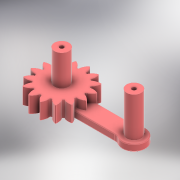
# Autodesk Inventor part: BRAÇO ROBÓTICO - Garra A2a
Saved by Autodesk Inventor 2021 (Build 250183000, 183)
## iProperties
Created: 2020-08-23
Part Number: BRAÇO ROBÓTICO - Garra A2a
Material: Plástico PC/ABS
Document SubType Name: Modeling
Designer: Araújo, I.
Density: 0.357273 g/cm^3
Appearance: Liso - Branco
Mass: 0.693061 g
Surface Area: 18.6744 cm^2
Volume: 1.93987 cm^3
Author: Araújo, I.
## iProperties of the stored document _3DPrint.ipt
Created: 2020-11-23
Part Number: _3DPrint
Material: Genérico
Document SubType Name: Modeling
Designer: Araújo, I.
Mass: 1.93987 g
Surface Area: 18.6744 cm^2
Volume: 1.93987 cm^3
Density: 1 g/cm^3
Appearance: Padrão
Author: Araújo, I.
Autodesk Inventor part; units mm, degrees
ref_plane "YZ Plane" through (0, 0, 0) normal (1, 0, 0) x (0, 1, 0)
ref_plane "XZ Plane" through (0, 0, 0) normal (0, 1, 0) x (-1, 0, 0)
ref_plane "XY Plane" through (0, 0, 0) normal (0, 0, 1) x (1, 0, 0)
sketch "Esboço2" plane through (0, 0, 0) normal (0, 1, 0) x (-1, 0, 0)
  arc A0 (-2.0603, -3.4286) -> (-2.0603, 3.4286) centre (0, 0) ccw
  arc A1 (-22.9397, 3.4286) -> (-22.9397, -3.4286) centre (-25, 0) ccw
  line L0 (-3.6056, -3) -> (-21.3944, -3)
  line L1 (-3.6056, 3) -> (-21.3944, 3)
  arc A2 (-2.0603, -3.4286) -> (-3.6056, -3) centre (-3.6056, -6) ccw
  arc A3 (-3.6056, 3) -> (-2.0603, 3.4286) centre (-3.6056, 6) ccw
  arc A4 (-21.3944, -3) -> (-22.9397, -3.4286) centre (-21.3944, -6) ccw
  arc A5 (-22.9397, 3.4286) -> (-21.3944, 3) centre (-21.3944, 6) ccw
  dimension "d64" = 6
  dimension "d65" = 3
  dimension "d94" = 25
  dimension "d95" = 4
  constraints: 12 point on circle, 8 tangent, 6 centre point, 4 end point, 4 equal radius, 2 parallel, 1 coincident, 1 horizontal, 1 horizontal alignment
  measures "d64" distance between parallel lines of L1 L0
  measures "d65" radius of A2
  measures "d94" distance of A1.centre A0.centre
  measures "d95" radius of A0
extrude "Extrusão2" add sketch "Esboço2" along normal blind 2.5
fillet "Arredondamento2" radius 0.3 16 edges at (22.1962, 2.5, 3.1091) (29, 2.5, 0) (22.1962, 2.5, -3.1091) (12.5, 2.5, -3) (2.8038, 2.5, -3.1091) (-4, 2.5, 0) (2.8038, 2.5, 3.1091) (12.5, 2.5, 3) (22.1962, 0, 3.1091) (29, 0, 0) (22.1962, 0, -3.1091) (12.5, 0, -3) (2.8038, 0, -3.1091) (-4, 0, 0) (2.8038, 0, 3.1091) (12.5, 0, 3)
sketch "Esboço1" plane through (0, 0, 0) normal (0, 1, 0) x (-1, 0, 0)
  circle A0 centre (0, 0) radius 8.5 construction
  line L0 (-16.1333, -15) -> (-23.1333, -15) construction
  line L1 (-23.1333, -15) -> (-23.1333, -7) construction
  line L2 (-23.1333, -7) -> (-16.1333, -7) construction
  line L3 (-16.1333, -7) -> (-16.1333, -15) construction
  circle A1 centre (0, 0) radius 9.6333
  circle A2 centre (0, 0) radius 7.3667 construction
  circle A3 centre (0, 0) radius 7.1778 construction
  line L4 (0, -15) -> (-1.1333, -15) construction
  line L5 (0, 0) -> (0, -9.6333)
  arc A4 (1.1679, -7.3143) -> (1.1647, -7.274) centre (0.3979, -7.3559) ccw construction
  line L6 (1.1647, -7.274) -> (0, 0) construction
  line L7 (0, 0) -> (0.3979, -7.3559) construction
  line L8 (0, 0) -> (-0.3731, -7.3572) construction
  line L9 (0, 0) -> (-1.1401, -7.2779) construction
  line L10 (0, 0) -> (-1.8946, -7.1189) construction
  line L11 (0, 0) -> (-2.6284, -6.8818) construction
  line L12 (1.1679, -7.3143) -> (0.3979, -7.3559) construction
  arc A5 (1.1665, -7.4353) -> (1.1679, -7.3143) centre (-0.3731, -7.3572) ccw construction
  line L13 (1.1665, -7.4353) -> (-0.3731, -7.3572) construction
  arc A6 (1.144, -7.6357) -> (1.1665, -7.4353) centre (-1.1401, -7.2779) ccw construction
  line L14 (1.144, -7.6357) -> (-1.1401, -7.2779) construction
  line L15 (-1.8946, -7.1189) -> (1.084, -7.9116) construction
  line L16 (-2.6284, -6.8818) -> (0.9706, -8.2564) construction
  arc A7 (1.084, -7.9116) -> (1.144, -7.6357) centre (-1.8946, -7.1189) ccw construction
  arc A8 (0.9706, -8.2564) -> (1.084, -7.9116) centre (-2.6284, -6.8818) ccw construction
  line L17 (0, 0) -> (-3.3333, -6.5694) construction
  line L18 (0, 0) -> (-4.0018, -6.185) construction
  line L19 (0, 0) -> (-4.6263, -5.7328) construction
  line L20 (-3.3333, -6.5694) -> (0.7891, -8.6611) construction
  line L21 (-4.0018, -6.185) -> (0.5261, -9.1145) construction
  line L22 (-4.6263, -5.7328) -> (0.1698, -9.6033) construction
  arc A9 (0.7891, -8.6611) -> (0.9706, -8.2564) centre (-3.3333, -6.5694) ccw construction
  arc A10 (0.5261, -9.1145) -> (0.7891, -8.6611) centre (-4.0018, -6.185) ccw construction
  arc A11 (0.1698, -9.6033) -> (0.5261, -9.1145) centre (-4.6263, -5.7328) ccw construction
  line L23 (0, 0) -> (-5.2002, -5.2178) construction
  line L24 (-5.2002, -5.2178) -> (-0.2895, -10.1121) construction
  arc A12 (-0.2895, -10.1121) -> (0.1698, -9.6033) centre (-5.2002, -5.2178) ccw construction
  line L25 (0, 0) -> (-5.7172, -4.6456) construction
  line L26 (-5.7172, -4.6456) -> (-0.8592, -10.6241) construction
  arc A13 (-0.8592, -10.6241) -> (-0.2895, -10.1121) centre (-5.7172, -4.6456) ccw construction
  spline S0 degree 4 poles (1.1647, -7.274) (1.1686, -7.2985) (1.1736, -7.4195) (1.154, -7.6223) (1.0788, -7.957) (0.9627, -8.2995) (0.7787, -8.7043) (0.3958, -9.356) (-0.0581, -9.9105) (-0.4987, -10.3319) (-0.8592, -10.6241) knots 0 0 0 0 0 0.136483 0.216899 0.310564 0.415677 0.531051 0.655814 1 1 1 1 1
  line L27 (0, 0) -> (0.8885, -8.4534) construction
  line L28 (0, -19.8966) -> (0, 14.3795) projected
  line L29 (-1.1333, -15) -> (-16.1333, -15) construction
  spline S1 degree 4 poles (-1.1647, -7.274) (-1.1686, -7.2985) (-1.1736, -7.4195) (-1.154, -7.6223) (-1.0788, -7.957) (-0.9627, -8.2995) (-0.7787, -8.7043) (-0.3958, -9.356) (0.0581, -9.9105) (0.4987, -10.3319) (0.8592, -10.6241) knots 0 0 0 0 0 0.136483 0.216899 0.310564 0.415677 0.531051 0.655814 1 1 1 1 1
  arc A14 (-1.6676, -6.9814) -> (-1.3161, -7.0561) centre (0, 0) ccw
  arc A15 (-1.1647, -7.274) -> (-1.3161, -7.0561) centre (-1.3508, -7.2418) ccw
  arc A16 (-1.6676, -6.9814) -> (-1.8946, -7.1189) centre (-1.7115, -7.1651) ccw
  spline S2 degree 4 poles (4.0226, -6.1714) (4.0362, -6.1922) (4.0899, -6.3007) (4.1545, -6.4939) (4.2219, -6.8302) (4.2552, -7.1904) (4.2517, -7.6351) (4.1671, -8.3862) (3.9779, -9.0773) (3.7468, -9.6415) (3.5363, -10.0551) knots 0 0 0 0 0 0.136483 0.216899 0.310564 0.415677 0.531051 0.655814 1 1 1 1 1
  spline S3 degree 4 poles (1.8946, -7.1189) (1.9009, -7.1428) (1.9457, -7.2554) (2.046, -7.4327) (2.2508, -7.7078) (2.4962, -7.9736) (2.829, -8.2685) (3.4438, -8.7082) (4.084, -9.03) (4.6579, -9.2358) (5.1061, -9.3561) knots 0 0 0 0 0 0.136483 0.216899 0.310564 0.415677 0.531051 0.655814 1 1 1 1 1
  spline S4 degree 4 poles (6.185, -4.0018) (6.2058, -4.0152) (6.2991, -4.0925) (6.4366, -4.2427) (6.635, -4.5225) (6.8119, -4.838) (6.9896, -5.2457) (7.2178, -5.9663) (7.326, -6.6746) (7.3444, -7.284) (7.3203, -7.7474) knots 0 0 0 0 0 0.136483 0.216899 0.310564 0.415677 0.531051 0.655814 1 1 1 1 1
  spline S5 degree 4 poles (4.6263, -5.7328) (4.6418, -5.7521) (4.7285, -5.8368) (4.8923, -5.9579) (5.1913, -6.126) (5.5236, -6.2689) (5.9475, -6.403) (6.688, -6.5546) (7.4038, -6.5882) (8.0118, -6.5428) (8.4702, -6.4704) knots 0 0 0 0 0 0.136483 0.216899 0.310564 0.415677 0.531051 0.655814 1 1 1 1 1
  spline S6 degree 4 poles (7.2779, -1.1401) (7.3024, -1.1439) (7.419, -1.1766) (7.6058, -1.2579) (7.9009, -1.4328) (8.1908, -1.6491) (8.5189, -1.9492) (9.0204, -2.5147) (9.4075, -3.1177) (9.6721, -3.667) (9.8386, -4.1002) knots 0 0 0 0 0 0.136483 0.216899 0.310564 0.415677 0.531051 0.655814 1 1 1 1 1
  spline S7 degree 4 poles (6.5581, -3.3554) (6.5801, -3.3668) (6.6937, -3.4089) (6.8926, -3.4529) (7.2341, -3.4849) (7.5958, -3.4803) (8.0377, -3.4303) (8.7758, -3.2676) (9.4434, -3.0073) (9.9803, -2.7184) (10.3696, -2.4659) knots 0 0 0 0 0 0.136483 0.216899 0.310564 0.415677 0.531051 0.655814 1 1 1 1 1
  spline S8 degree 4 poles (7.1124, 1.9186) (7.1363, 1.9251) (7.2562, 1.9427) (7.4599, 1.9444) (7.8006, 1.9046) (8.1534, 1.825) (8.5752, 1.6842) (9.2634, 1.3716) (9.8622, 0.9782) (10.3274, 0.584) (10.6557, 0.256) knots 0 0 0 0 0 0.136483 0.216899 0.310564 0.415677 0.531051 0.655814 1 1 1 1 1
  spline S9 degree 4 poles (7.3559, -0.3979) (7.3806, -0.3993) (7.5015, -0.3916) (7.7011, -0.3509) (8.0261, -0.2412) (8.3547, -0.0899) (8.738, 0.1355) (9.3462, 0.5843) (9.8501, 1.0937) (10.2232, 1.5759) (10.4761, 1.965) knots 0 0 0 0 0 0.136483 0.216899 0.310564 0.415677 0.531051 0.655814 1 1 1 1 1
  spline S10 degree 4 poles (5.7172, 4.6456) (5.7363, 4.6613) (5.8387, 4.7261) (6.0241, 4.8105) (6.3515, 4.9128) (6.7062, 4.9835) (7.1488, 5.0265) (7.9047, 5.0208) (8.6118, 4.9049) (9.197, 4.7341) (9.6303, 4.568) knots 0 0 0 0 0 0.136483 0.216899 0.310564 0.415677 0.531051 0.655814 1 1 1 1 1
  spline S11 degree 4 poles (6.8818, 2.6284) (6.905, 2.6372) (7.0123, 2.6934) (7.1781, 2.8117) (7.4303, 3.0442) (7.669, 3.316) (7.9275, 3.6778) (8.3005, 4.3352) (8.5537, 5.0055) (8.6983, 5.5978) (8.7711, 6.0561) knots 0 0 0 0 0 0.136483 0.216899 0.310564 0.415677 0.531051 0.655814 1 1 1 1 1
  spline S12 degree 4 poles (3.3333, 6.5694) (3.3445, 6.5915) (3.4116, 6.6923) (3.5467, 6.8448) (3.8042, 7.0714) (4.0995, 7.2803) (4.4863, 7.4996) (5.1791, 7.8019) (5.8722, 7.9836) (6.4764, 8.0656) (6.9398, 8.09) knots 0 0 0 0 0 0.136483 0.216899 0.310564 0.415677 0.531051 0.655814 1 1 1 1 1
  spline S13 degree 4 poles (5.2178, 5.2002) (5.2354, 5.2177) (5.3105, 5.3127) (5.4139, 5.4882) (5.5498, 5.8032) (5.6572, 6.1486) (5.7462, 6.5842) (5.8196, 7.3365) (5.7782, 8.0519) (5.6695, 8.6518) (5.5496, 9.1001) knots 0 0 0 0 0 0.136483 0.216899 0.310564 0.415677 0.531051 0.655814 1 1 1 1 1
  spline S14 degree 4 poles (0.3731, 7.3572) (0.3743, 7.382) (0.3947, 7.5014) (0.456, 7.6956) (0.5991, 8.0074) (0.7839, 8.3183) (1.0481, 8.676) (1.5581, 9.2339) (2.1173, 9.6818) (2.6359, 10.0024) (3.0493, 10.2133) knots 0 0 0 0 0 0.136483 0.216899 0.310564 0.415677 0.531051 0.655814 1 1 1 1 1
  spline S15 degree 4 poles (2.6516, 6.8729) (2.6605, 6.896) (2.6905, 7.0134) (2.7135, 7.2158) (2.7096, 7.5588) (2.6672, 7.918) (2.5714, 8.3522) (2.3324, 9.0693) (2.0037, 9.706) (1.6603, 10.2098) (1.3684, 10.5706) knots 0 0 0 0 0 0.136483 0.216899 0.310564 0.415677 0.531051 0.655814 1 1 1 1 1
  spline S16 degree 4 poles (-2.6516, 6.8729) (-2.6605, 6.896) (-2.6905, 7.0134) (-2.7135, 7.2158) (-2.7096, 7.5588) (-2.6672, 7.918) (-2.5714, 8.3522) (-2.3324, 9.0693) (-2.0037, 9.706) (-1.6603, 10.2098) (-1.3684, 10.5706) knots 0 0 0 0 0 0.136483 0.216899 0.310564 0.415677 0.531051 0.655814 1 1 1 1 1
  spline S17 degree 4 poles (-0.3731, 7.3572) (-0.3743, 7.382) (-0.3947, 7.5014) (-0.456, 7.6956) (-0.5991, 8.0074) (-0.7839, 8.3183) (-1.0481, 8.676) (-1.5581, 9.2339) (-2.1173, 9.6818) (-2.6359, 10.0024) (-3.0493, 10.2133) knots 0 0 0 0 0 0.136483 0.216899 0.310564 0.415677 0.531051 0.655814 1 1 1 1 1
  spline S18 degree 4 poles (-5.2178, 5.2002) (-5.2354, 5.2177) (-5.3105, 5.3127) (-5.4139, 5.4882) (-5.5498, 5.8032) (-5.6572, 6.1486) (-5.7462, 6.5842) (-5.8196, 7.3365) (-5.7782, 8.0519) (-5.6695, 8.6518) (-5.5496, 9.1001) knots 0 0 0 0 0 0.136483 0.216899 0.310564 0.415677 0.531051 0.655814 1 1 1 1 1
  spline S19 degree 4 poles (-3.3333, 6.5694) (-3.3445, 6.5915) (-3.4116, 6.6923) (-3.5467, 6.8448) (-3.8042, 7.0714) (-4.0995, 7.2803) (-4.4863, 7.4996) (-5.1791, 7.8019) (-5.8722, 7.9836) (-6.4764, 8.0656) (-6.9398, 8.09) knots 0 0 0 0 0 0.136483 0.216899 0.310564 0.415677 0.531051 0.655814 1 1 1 1 1
  spline S20 degree 4 poles (-6.8818, 2.6284) (-6.905, 2.6372) (-7.0123, 2.6934) (-7.1781, 2.8117) (-7.4303, 3.0442) (-7.669, 3.316) (-7.9275, 3.6778) (-8.3005, 4.3352) (-8.5537, 5.0055) (-8.6983, 5.5978) (-8.7711, 6.0561) knots 0 0 0 0 0 0.136483 0.216899 0.310564 0.415677 0.531051 0.655814 1 1 1 1 1
  spline S21 degree 4 poles (-5.7172, 4.6456) (-5.7363, 4.6613) (-5.8387, 4.7261) (-6.0241, 4.8105) (-6.3515, 4.9128) (-6.7062, 4.9835) (-7.1488, 5.0265) (-7.9047, 5.0208) (-8.6118, 4.9049) (-9.197, 4.7341) (-9.6303, 4.568) knots 0 0 0 0 0 0.136483 0.216899 0.310564 0.415677 0.531051 0.655814 1 1 1 1 1
  spline S22 degree 4 poles (-7.3559, -0.3979) (-7.3806, -0.3993) (-7.5015, -0.3916) (-7.7011, -0.3509) (-8.0261, -0.2412) (-8.3547, -0.0899) (-8.738, 0.1355) (-9.3462, 0.5843) (-9.8501, 1.0937) (-10.2232, 1.5759) (-10.4761, 1.965) knots 0 0 0 0 0 0.136483 0.216899 0.310564 0.415677 0.531051 0.655814 1 1 1 1 1
  spline S23 degree 4 poles (-7.1124, 1.9186) (-7.1363, 1.9251) (-7.2562, 1.9427) (-7.4599, 1.9444) (-7.8006, 1.9046) (-8.1534, 1.825) (-8.5752, 1.6842) (-9.2634, 1.3716) (-9.8622, 0.9782) (-10.3274, 0.584) (-10.6557, 0.256) knots 0 0 0 0 0 0.136483 0.216899 0.310564 0.415677 0.531051 0.655814 1 1 1 1 1
  spline S24 degree 4 poles (-6.5581, -3.3554) (-6.5801, -3.3668) (-6.6937, -3.4089) (-6.8926, -3.4529) (-7.2341, -3.4849) (-7.5958, -3.4803) (-8.0377, -3.4303) (-8.7758, -3.2676) (-9.4434, -3.0073) (-9.9803, -2.7184) (-10.3696, -2.4659) knots 0 0 0 0 0 0.136483 0.216899 0.310564 0.415677 0.531051 0.655814 1 1 1 1 1
  spline S25 degree 4 poles (-7.2779, -1.1401) (-7.3024, -1.1439) (-7.419, -1.1766) (-7.6058, -1.2579) (-7.9009, -1.4328) (-8.1908, -1.6491) (-8.5189, -1.9492) (-9.0204, -2.5147) (-9.4075, -3.1177) (-9.6721, -3.667) (-9.8386, -4.1002) knots 0 0 0 0 0 0.136483 0.216899 0.310564 0.415677 0.531051 0.655814 1 1 1 1 1
  spline S26 degree 4 poles (-4.6263, -5.7328) (-4.6418, -5.7521) (-4.7285, -5.8368) (-4.8923, -5.9579) (-5.1913, -6.126) (-5.5236, -6.2689) (-5.9475, -6.403) (-6.688, -6.5546) (-7.4038, -6.5882) (-8.0118, -6.5428) (-8.4702, -6.4704) knots 0 0 0 0 0 0.136483 0.216899 0.310564 0.415677 0.531051 0.655814 1 1 1 1 1
  spline S27 degree 4 poles (-6.185, -4.0018) (-6.2058, -4.0152) (-6.2991, -4.0925) (-6.4366, -4.2427) (-6.635, -4.5225) (-6.8119, -4.838) (-6.9896, -5.2457) (-7.2178, -5.9663) (-7.326, -6.6746) (-7.3444, -7.284) (-7.3203, -7.7474) knots 0 0 0 0 0 0.136483 0.216899 0.310564 0.415677 0.531051 0.655814 1 1 1 1 1
  spline S28 degree 4 poles (-1.8946, -7.1189) (-1.9009, -7.1428) (-1.9457, -7.2554) (-2.046, -7.4327) (-2.2508, -7.7078) (-2.4962, -7.9736) (-2.829, -8.2685) (-3.4438, -8.7082) (-4.084, -9.03) (-4.6579, -9.2358) (-5.1061, -9.3561) knots 0 0 0 0 0 0.136483 0.216899 0.310564 0.415677 0.531051 0.655814 1 1 1 1 1
  spline S29 degree 4 poles (-4.0226, -6.1714) (-4.0362, -6.1922) (-4.0899, -6.3007) (-4.1545, -6.4939) (-4.2219, -6.8302) (-4.2552, -7.1904) (-4.2517, -7.6351) (-4.1671, -8.3862) (-3.9779, -9.0773) (-3.7468, -9.6415) (-3.5363, -10.0551) knots 0 0 0 0 0 0.136483 0.216899 0.310564 0.415677 0.531051 0.655814 1 1 1 1 1
  arc A17 (1.8946, -7.1189) -> (1.6676, -6.9814) centre (1.7115, -7.1651) ccw
  arc A18 (1.3161, -7.0561) -> (1.6676, -6.9814) centre (0, 0) ccw
  arc A19 (1.3161, -7.0561) -> (1.1647, -7.274) centre (1.3508, -7.2418) ccw
  arc A20 (4.6263, -5.7328) -> (4.363, -5.6995) centre (4.4778, -5.8495) ccw
  arc A21 (4.0723, -5.9107) -> (4.363, -5.6995) centre (0, 0) ccw
  arc A22 (4.0723, -5.9107) -> (4.0226, -6.1714) centre (4.1795, -6.0663) ccw
  arc A23 (6.5581, -3.3554) -> (6.304, -3.4322) centre (6.4699, -3.5225) ccw
  arc A24 (6.1244, -3.7434) -> (6.304, -3.4322) centre (0, 0) ccw
  arc A25 (6.1244, -3.7434) -> (6.185, -4.0018) centre (6.2855, -3.8419) ccw
  arc A26 (7.3559, -0.3979) -> (7.155, -0.5714) centre (7.3433, -0.5864) ccw
  arc A27 (7.1174, -0.9287) -> (7.155, -0.5714) centre (0, 0) ccw
  arc A28 (7.1174, -0.9287) -> (7.2779, -1.1401) centre (7.3047, -0.9532) ccw
  arc A29 (6.8818, 2.6284) -> (6.7688, 2.3882) centre (6.9469, 2.4511) ccw
  arc A30 (6.8799, 2.0465) -> (6.7688, 2.3882) centre (0, 0) ccw
  arc A31 (6.8799, 2.0465) -> (7.1124, 1.9186) centre (7.0609, 2.1003) ccw
  arc A32 (5.2178, 5.2002) -> (5.2122, 4.9349) centre (5.3494, 5.0648) ccw
  arc A33 (5.4527, 4.6678) -> (5.2122, 4.9349) centre (0, 0) ccw
  arc A34 (5.4527, 4.6678) -> (5.7172, 4.6456) centre (5.5962, 4.7907) ccw
  arc A35 (2.6516, 6.8729) -> (2.7544, 6.6282) centre (2.8269, 6.8027) ccw
  arc A36 (3.0827, 6.4821) -> (2.7544, 6.6282) centre (0, 0) ccw
  arc A37 (3.0827, 6.4821) -> (3.3333, 6.5694) centre (3.1638, 6.6527) ccw
  arc A38 (-0.3731, 7.3572) -> (-0.1797, 7.1755) centre (-0.1844, 7.3644) ccw
  arc A39 (0.1797, 7.1755) -> (-0.1797, 7.1755) centre (0, 0) ccw
  arc A40 (0.1797, 7.1755) -> (0.3731, 7.3572) centre (0.1844, 7.3644) ccw
  arc A41 (-3.3333, 6.5694) -> (-3.0827, 6.4821) centre (-3.1638, 6.6527) ccw
  arc A42 (-2.7544, 6.6282) -> (-3.0827, 6.4821) centre (0, 0) ccw
  arc A43 (-2.7544, 6.6282) -> (-2.6516, 6.8729) centre (-2.8269, 6.8027) ccw
  arc A44 (-5.7172, 4.6456) -> (-5.4527, 4.6678) centre (-5.5962, 4.7907) ccw
  arc A45 (-5.2122, 4.9349) -> (-5.4527, 4.6678) centre (0, 0) ccw
  arc A46 (-5.2122, 4.9349) -> (-5.2178, 5.2002) centre (-5.3494, 5.0648) ccw
  arc A47 (-7.1124, 1.9186) -> (-6.8799, 2.0465) centre (-7.0609, 2.1003) ccw
  arc A48 (-6.7688, 2.3882) -> (-6.8799, 2.0465) centre (0, 0) ccw
  arc A49 (-6.7688, 2.3882) -> (-6.8818, 2.6284) centre (-6.9469, 2.4511) ccw
  arc A50 (-7.2779, -1.1401) -> (-7.1174, -0.9287) centre (-7.3047, -0.9532) ccw
  arc A51 (-7.155, -0.5714) -> (-7.1174, -0.9287) centre (0, 0) ccw
  arc A52 (-7.155, -0.5714) -> (-7.3559, -0.3979) centre (-7.3433, -0.5864) ccw
  arc A53 (-6.185, -4.0018) -> (-6.1244, -3.7434) centre (-6.2855, -3.8419) ccw
  arc A54 (-6.304, -3.4322) -> (-6.1244, -3.7434) centre (0, 0) ccw
  arc A55 (-6.304, -3.4322) -> (-6.5581, -3.3554) centre (-6.4699, -3.5225) ccw
  arc A56 (-4.0226, -6.1714) -> (-4.0723, -5.9107) centre (-4.1795, -6.0663) ccw
  arc A57 (-4.363, -5.6995) -> (-4.0723, -5.9107) centre (0, 0) ccw
  arc A58 (-4.363, -5.6995) -> (-4.6263, -5.7328) centre (-4.4778, -5.8495) ccw
  point P0 (-1.1679, -7.3143)
  point P1 (-1.1665, -7.4353)
  point P2 (-1.144, -7.6357)
  point P3 (-1.084, -7.9116)
  point P4 (-0.9706, -8.2564)
  point P5 (-0.7891, -8.6611)
  point P6 (-0.5261, -9.1145)
  point P7 (-0.1698, -9.6033)
  point P8 (0.2895, -10.1121)
  point P9 (-0.1462, -9.6322)
  point P10 (0.1462, -9.6322)
  point P11 (4.0419, -6.2069)
  point P12 (4.0899, -6.318)
  point P13 (4.1508, -6.5103)
  point P14 (4.2082, -6.7867)
  point P15 (4.2449, -7.1478)
  point P16 (4.2437, -7.5914)
  point P17 (4.1878, -8.1126)
  point P18 (4.0611, -8.7039)
  point P19 (3.8485, -9.3556)
  point P20 (4.25, -7.3612)
  point P21 (1.9081, -7.1569)
  point P22 (1.9585, -7.2669)
  point P23 (2.0606, -7.4409)
  point P24 (2.2277, -7.6685)
  point P25 (2.4715, -7.9374)
  point P26 (2.8019, -8.2333)
  point P27 (3.2266, -8.5405)
  point P28 (3.7509, -8.8421)
  point P29 (4.3774, -9.1201)
  point P30 (6.217, -4.0263)
  point P31 (6.3061, -4.1083)
  point P32 (6.44, -4.2591)
  point P33 (6.6048, -4.4883)
  point P34 (6.7851, -4.8033)
  point P35 (6.9645, -5.209)
  point P36 (7.1254, -5.7079)
  point P37 (7.2502, -6.2996)
  point P38 (7.321, -6.9814)
  point P39 (6.8766, -4.9962)
  point P40 (4.6541, -5.7621)
  point P41 (4.745, -5.8421)
  point P42 (4.909, -5.9595)
  point P43 (5.1541, -6.0994)
  point P44 (5.4862, -6.2459)
  point P45 (5.9085, -6.3818)
  point P46 (6.4214, -6.4898)
  point P47 (7.023, -6.552)
  point P48 (7.7084, -6.5512)
  point P49 (7.3172, -1.1495)
  point P50 (7.4319, -1.1882)
  point P51 (7.6155, -1.2715)
  point P52 (7.8593, -1.4139)
  point P53 (8.1522, -1.6283)
  point P54 (8.4811, -1.926)
  point P55 (8.831, -2.3162)
  point P56 (9.1857, -2.8061)
  point P57 (9.5277, -3.4001)
  point P58 (8.3143, -1.7672)
  point P59 (6.5954, -3.371)
  point P60 (6.7109, -3.4071)
  point P61 (6.9085, -3.4476)
  point P62 (7.1894, -3.4757)
  point P63 (7.5524, -3.4744)
  point P64 (7.9934, -3.4269)
  point P65 (8.5059, -3.3169)
  point P66 (9.0808, -3.1291)
  point P67 (9.7066, -2.8495)
  point P68 (7.1521, 1.926)
  point P69 (7.2726, 1.9373)
  point P70 (7.4743, 1.9359)
  point P71 (7.755, 1.905)
  point P72 (8.1097, 1.8283)
  point P73 (8.5312, 1.6901)
  point P74 (9.0096, 1.4759)
  point P75 (9.5329, 1.1727)
  point P76 (10.0869, 0.7691)
  point P77 (8.3143, 1.7672)
  point P78 (7.3963, -0.3969)
  point P79 (7.5165, -0.3829)
  point P80 (7.7135, -0.3396)
  point P81 (7.9816, -0.251)
  point P82 (8.3126, -0.1022)
  point P83 (8.6962, 0.1206)
  point P84 (9.1196, 0.4295)
  point P85 (9.5684, 0.8349)
  point P86 (10.0264, 1.3449)
  point P87 (5.7504, 4.6686)
  point P88 (5.8559, 4.7279)
  point P89 (6.0407, 4.8086)
  point P90 (6.3097, 4.8945)
  point P91 (6.6649, 4.9687)
  point P92 (7.1062, 5.0139)
  point P93 (7.6304, 5.0129)
  point P94 (8.2318, 4.9487)
  point P95 (8.902, 4.8054)
  point P96 (6.8766, 4.9962)
  point P97 (6.9183, 2.6457)
  point P98 (7.0224, 2.7074)
  point P99 (7.1847, 2.8271)
  point P100 (7.3936, 3.017)
  point P101 (7.6355, 3.2876)
  point P102 (7.8953, 3.6472)
  point P103 (8.1564, 4.1017)
  point P104 (8.4016, 4.6546)
  point P105 (8.6126, 5.3067)
  point P106 (3.3544, 6.6038)
  point P107 (3.4266, 6.7009)
  point P108 (3.5626, 6.8499)
  point P109 (3.7734, 7.0378)
  point P110 (4.0678, 7.2501)
  point P111 (4.4525, 7.4708)
  point P112 (4.9318, 7.683)
  point P113 (5.5073, 7.869)
  point P114 (6.1779, 8.0107)
  point P115 (4.25, 7.3612)
  point P116 (5.2441, 5.2309)
  point P117 (5.3141, 5.3296)
  point P118 (5.4137, 5.505)
  point P119 (5.5273, 5.7635)
  point P120 (5.6382, 6.1091)
  point P121 (5.7293, 6.5432)
  point P122 (5.783, 7.0646)
  point P123 (5.782, 7.6694)
  point P124 (5.7095, 8.351)
  point P125 (0.3784, 7.3972)
  point P126 (0.4049, 7.5154)
  point P127 (0.4685, 7.7067)
  point P128 (0.5846, 7.9641)
  point P129 (0.7672, 8.2778)
  point P130 (1.0289, 8.6359)
  point P131 (1.3804, 9.0247)
  point P132 (1.8305, 9.4287)
  point P133 (2.3855, 9.8309)
  point P134 (0.8885, 8.4534)
  point P135 (2.6631, 6.9116)
  point P136 (2.6869, 7.0303)
  point P137 (2.7066, 7.231)
  point P138 (2.7052, 7.5133)
  point P139 (2.666, 7.8742)
  point P140 (2.5726, 8.3078)
  point P141 (2.4096, 8.806)
  point P142 (2.1627, 9.3581)
  point P143 (1.8193, 9.9513)
  point P144 (-2.6631, 6.9116)
  point P145 (-2.6869, 7.0303)
  point P146 (-2.7066, 7.231)
  point P147 (-2.7052, 7.5133)
  point P148 (-2.666, 7.8742)
  point P149 (-2.5726, 8.3078)
  point P150 (-2.4096, 8.806)
  point P151 (-2.1627, 9.3581)
  point P152 (-1.8193, 9.9513)
  point P153 (-2.6266, 8.084)
  point P154 (-0.3784, 7.3972)
  point P155 (-0.4049, 7.5154)
  point P156 (-0.4685, 7.7067)
  point P157 (-0.5846, 7.9641)
  point P158 (-0.7672, 8.2778)
  point P159 (-1.0289, 8.6359)
  point P160 (-1.3804, 9.0247)
  point P161 (-1.8305, 9.4287)
  point P162 (-2.3855, 9.8309)
  point P163 (-5.2441, 5.2309)
  point P164 (-5.3141, 5.3296)
  point P165 (-5.4137, 5.505)
  point P166 (-5.5273, 5.7635)
  point P167 (-5.6382, 6.1091)
  point P168 (-5.7293, 6.5432)
  point P169 (-5.783, 7.0646)
  point P170 (-5.782, 7.6694)
  point P171 (-5.7095, 8.351)
  point P172 (-5.6876, 6.3167)
  point P173 (-3.3544, 6.6038)
  point P174 (-3.4266, 6.7009)
  point P175 (-3.5626, 6.8499)
  point P176 (-3.7734, 7.0378)
  point P177 (-4.0678, 7.2501)
  point P178 (-4.4525, 7.4708)
  point P179 (-4.9318, 7.683)
  point P180 (-5.5073, 7.869)
  point P181 (-6.1779, 8.0107)
  point P182 (-6.9183, 2.6457)
  point P183 (-7.0224, 2.7074)
  point P184 (-7.1847, 2.8271)
  point P185 (-7.3936, 3.017)
  point P186 (-7.6355, 3.2876)
  point P187 (-7.8953, 3.6472)
  point P188 (-8.1564, 4.1017)
  point P189 (-8.4016, 4.6546)
  point P190 (-8.6126, 5.3067)
  point P191 (-7.7651, 3.4573)
  point P192 (-5.7504, 4.6686)
  point P193 (-5.8559, 4.7279)
  point P194 (-6.0407, 4.8086)
  point P195 (-6.3097, 4.8945)
  point P196 (-6.6649, 4.9687)
  point P197 (-7.1062, 5.0139)
  point P198 (-7.6304, 5.0129)
  point P199 (-8.2318, 4.9487)
  dimension "d13" = 17
  dimension "d23" = 19.2667
  dimension "d25" = 14.7333
  dimension "d24" = 1.1333
  dimension "d46" = 6
  dimension "d47" = 6
  dimension "d48" = 6
  dimension "d49" = 6
  dimension "d51" = 6
  dimension "d52" = 6
  dimension "d53" = 6
  dimension "d54" = 6
  dimension "d56" = 0.1889
  dimension "d57" = 6
  dimension "d67" = 15
  dimension "d68" = 0
  dimension "d69" = 15
  dimension "d70" = 8
  dimension "d71" = 7
  dimension "d73" = 6
  dimension "d74" = 6
  dimension "d85" = 360
  dimension "d89" = 360
  constraints: 112 point on circle, 56 centre point, 50 end point, 19 coincident, 11 symmetric about line, 10 perpendicular, 3 horizontal, 2 tangent, 1 concentric, 1 vertical alignment, 893 other
  measures "d24" distance of L4.start L4.end
  measures "d46" angle of L8 L7
  measures "d47" angle of L9 L8
  measures "d48" angle of L10 L9
  measures "d49" angle of L11 L10
  measures "d51" angle of L17 L11
  measures "d52" angle of L18 L17
  measures "d53" angle of L19 L18
  measures "d54" angle of L23 L19
  measures "d57" angle of L25 L23
  measures "d67" distance from line of point (0, 0) L4
  measures "d68" distance between parallel lines of L28 L5
  measures "d69" distance of L4.end L29.end
  measures "d70" distance of L0.end L1.end
  measures "d71" distance of L1.end L2.end
  measures "d73" angle of L5 L27
  measures "d74" angle of L7 L6
extrude "Extrusão1" add sketch "Esboço1" along normal blind 5.5 contours S9 A26 A27 A28 S6 A1 S7 A23 A24 A25 S4 S5 A20 A21 A22 S2 S3 A17 A18 A19 S0 L5 L28 A39 A40 S14 S15 A35 A36 A37 S12 S13 A32 A33 A34 S10 S11 A29 A30 A31 S8 | A1 S1 A15 A14 A16 S28 S29 A56 A57 A58 S26 S27 A53 A54 A55 S24 S25 A50 A51 A52 S22 S23 A47 A48 A49 S20 S21 A44 A45 A46 S18 S19 A41 A42 A43 S16 S17 A38 A39 L28 L5
sketch "Esboço3" plane through (0, 2.5, 0) normal (0, 1, 0) x (1, 0, 0)
  circle A0 centre (25, 0) radius 2.5
  circle A1 centre (0, 0) radius 2.5
  arc A2 (23.0942, -3.1714) -> (23.0942, 3.1714) centre (25, 0) ccw projected
  arc A3 (-7.1174, 0.9287) -> (-7.155, 0.5714) centre (0, 0) ccw projected
  dimension "d97" = 5
  constraints: 2 centre point, 2 coincident, 1 equal radius
  measures "d97" diameter of A0
extrude "Extrusão3" add sketch "Esboço3" along normal blind 13.7
sketch "Esboço4" plane through (0, 16.2, 0) normal (0, 1, 0) x (1, 0, 0)
  circle A0 centre (0, 0) radius 2.5 projected
  circle A1 centre (25, 0) radius 2.5 projected
  constraints: 2 coincident
hole "Furo1" at (0, 16.2, 0) at (25, 16.2, 0) direction (0, -1, 0) diameter 1.5 depth 10 tip angle 118
sketch "Esboço5" plane through (0, 0, 0) normal (0, -1, 0) x (1, 0, 0)
  line L0 (-0.05, 2.2995) -> (-0.391, 2.6715)
  line L1 (0.391, 2.6715) -> (0.05, 2.2995)
  arc A0 (0.05, 2.2995) -> (-0.05, 2.2995) centre (0, 0) ccw
  arc A1 (-7.155, -0.5714) -> (-7.1174, -0.9287) centre (0, 0) ccw projected
  circle A2 centre (0, 0) radius 2.7
  line L2 (0.663, 2.2024) -> (0.4537, 2.6616)
  arc A3 (0.7581, 2.1715) -> (0.663, 2.2024) centre (0, 0) ccw
  line L3 (1.1974, 2.42) -> (0.7581, 2.1715)
  line L4 (1.3111, 1.8897) -> (1.254, 2.3911)
  arc A4 (1.392, 1.8309) -> (1.3111, 1.8897) centre (0, 0) ccw
  line L5 (1.8866, 1.9315) -> (1.392, 1.8309)
  line L6 (1.8309, 1.392) -> (1.9315, 1.8866)
  arc A5 (1.8897, 1.3111) -> (1.8309, 1.392) centre (0, 0) ccw
  line L7 (2.3911, 1.254) -> (1.8897, 1.3111)
  line L8 (2.1715, 0.7581) -> (2.42, 1.1974)
  arc A6 (2.2024, 0.663) -> (2.1715, 0.7581) centre (0, 0) ccw
  line L9 (2.6616, 0.4537) -> (2.2024, 0.663)
  line L10 (2.2995, 0.05) -> (2.6715, 0.391)
  arc A7 (2.2995, -0.05) -> (2.2995, 0.05) centre (0, 0) ccw
  line L11 (2.6715, -0.391) -> (2.2995, -0.05)
  line L12 (2.2024, -0.663) -> (2.6616, -0.4537)
  arc A8 (2.1715, -0.7581) -> (2.2024, -0.663) centre (0, 0) ccw
  line L13 (2.42, -1.1974) -> (2.1715, -0.7581)
  line L14 (1.8897, -1.3111) -> (2.3911, -1.254)
  arc A9 (1.8309, -1.392) -> (1.8897, -1.3111) centre (0, 0) ccw
  line L15 (1.9315, -1.8866) -> (1.8309, -1.392)
  line L16 (1.392, -1.8309) -> (1.8866, -1.9315)
  arc A10 (1.3111, -1.8897) -> (1.392, -1.8309) centre (0, 0) ccw
  line L17 (1.254, -2.3911) -> (1.3111, -1.8897)
  line L18 (0.7581, -2.1715) -> (1.1974, -2.42)
  arc A11 (0.663, -2.2024) -> (0.7581, -2.1715) centre (0, 0) ccw
  line L19 (0.4537, -2.6616) -> (0.663, -2.2024)
  line L20 (0.05, -2.2995) -> (0.391, -2.6715)
  arc A12 (-0.05, -2.2995) -> (0.05, -2.2995) centre (0, 0) ccw
  line L21 (-0.391, -2.6715) -> (-0.05, -2.2995)
  line L22 (-0.663, -2.2024) -> (-0.4537, -2.6616)
  arc A13 (-0.7581, -2.1715) -> (-0.663, -2.2024) centre (0, 0) ccw
  line L23 (-1.1974, -2.42) -> (-0.7581, -2.1715)
  line L24 (-1.3111, -1.8897) -> (-1.254, -2.3911)
  arc A14 (-1.392, -1.8309) -> (-1.3111, -1.8897) centre (0, 0) ccw
  line L25 (-1.8866, -1.9315) -> (-1.392, -1.8309)
  line L26 (-1.8309, -1.392) -> (-1.9315, -1.8866)
  arc A15 (-1.8897, -1.3111) -> (-1.8309, -1.392) centre (0, 0) ccw
  line L27 (-2.3911, -1.254) -> (-1.8897, -1.3111)
  line L28 (-2.1715, -0.7581) -> (-2.42, -1.1974)
  arc A16 (-2.2024, -0.663) -> (-2.1715, -0.7581) centre (0, 0) ccw
  line L29 (-2.6616, -0.4537) -> (-2.2024, -0.663)
  line L30 (-2.2995, -0.05) -> (-2.6715, -0.391)
  arc A17 (-2.2995, 0.05) -> (-2.2995, -0.05) centre (0, 0) ccw
  line L31 (-2.6715, 0.391) -> (-2.2995, 0.05)
  line L32 (-2.2024, 0.663) -> (-2.6616, 0.4537)
  arc A18 (-2.1715, 0.7581) -> (-2.2024, 0.663) centre (0, 0) ccw
  line L33 (-2.42, 1.1974) -> (-2.1715, 0.7581)
  line L34 (-1.8897, 1.3111) -> (-2.3911, 1.254)
  arc A19 (-1.8309, 1.392) -> (-1.8897, 1.3111) centre (0, 0) ccw
  line L35 (-1.9315, 1.8866) -> (-1.8309, 1.392)
  line L36 (-1.392, 1.8309) -> (-1.8866, 1.9315)
  arc A20 (-1.3111, 1.8897) -> (-1.392, 1.8309) centre (0, 0) ccw
  line L37 (-1.254, 2.3911) -> (-1.3111, 1.8897)
  line L38 (-0.7581, 2.1715) -> (-1.1974, 2.42)
  arc A21 (-0.663, 2.2024) -> (-0.7581, 2.1715) centre (0, 0) ccw
  line L39 (-0.4537, 2.6616) -> (-0.663, 2.2024)
  point P0 (0, 2.3)
  point P1 (0.7107, 2.1874)
  point P2 (1.3519, 1.8607)
  point P3 (1.8607, 1.3519)
  point P4 (2.1874, 0.7107)
  point P5 (2.3, 0)
  point P6 (2.1874, -0.7107)
  point P7 (1.8607, -1.3519)
  point P8 (1.3519, -1.8607)
  point P9 (0.7107, -2.1874)
  point P10 (0, -2.3)
  point P11 (-0.7107, -2.1874)
  point P12 (-1.3519, -1.8607)
  point P13 (-1.8607, -1.3519)
  point P14 (-2.1874, -0.7107)
  point P15 (-2.3, 0)
  point P16 (-2.1874, 0.7107)
  point P17 (-1.8607, 1.3519)
  point P18 (-1.3519, 1.8607)
  point P19 (-0.7107, 2.1874)
  point P20 (-0.4537, 2.6616)
  point P21 (-1.1974, 2.42)
  point P22 (-1.254, 2.3911)
  point P23 (-1.8866, 1.9315)
  point P24 (-1.9315, 1.8866)
  point P25 (-2.3911, 1.254)
  point P26 (-2.42, 1.1974)
  point P27 (-2.6616, 0.4537)
  point P28 (-2.6715, 0.391)
  point P29 (-2.6715, -0.391)
  point P30 (-2.6616, -0.4537)
  point P31 (-2.42, -1.1974)
  point P32 (-2.3911, -1.254)
  point P33 (-1.9315, -1.8866)
  point P34 (-1.8866, -1.9315)
  point P35 (-1.254, -2.3911)
  point P36 (-1.1974, -2.42)
  point P37 (-0.4537, -2.6616)
  point P38 (-0.391, -2.6715)
  point P39 (0.391, -2.6715)
  point P40 (0.4537, -2.6616)
  point P41 (1.1974, -2.42)
  point P42 (1.254, -2.3911)
  point P43 (1.8866, -1.9315)
  point P44 (1.9315, -1.8866)
  point P45 (2.3911, -1.254)
  point P46 (2.42, -1.1974)
  point P47 (2.6616, -0.4537)
  point P48 (2.6715, -0.391)
  point P49 (2.6715, 0.391)
  point P50 (2.6616, 0.4537)
  point P51 (2.42, 1.1974)
  point P52 (2.3911, 1.254)
  point P53 (1.9315, 1.8866)
  point P54 (1.8866, 1.9315)
  point P55 (1.254, 2.3911)
  point P56 (1.1974, 2.42)
  point P57 (0.4537, 2.6616)
  dimension "d113" = 5.4
  dimension "d109" = 85
  dimension "d111" = 0.1
  dimension "d115" = 2.3
  dimension "d118" = 360
  constraints: 80 end point, 41 point on circle, 20 centre point, 4 coincident, 1 equal length, 1 vertical alignment, 183 other
  measures "d109" angle of L1 L0
  measures "d111" distance of L1.end L0.start
  measures "d115" radius of A0
extrude "Extrusão4" cut sketch "Esboço5" against normal blind 3 contours A0 L1 A2 L2 A3 L3 L4 A4 L5 L6 A5 L7 L8 A6 L9 L10 A7 L11 L12 A8 L13 L14 A9 L15 L16 A10 L17 L18 A11 L19 L20 A12 L21 L22 A13 L23 L24 A14 L25 L26 A15 L27 L28 A16 L29 L30 A17 L31 L32 A18 L33 L34 A19 L35 L36 A20 L37 L38 A21 L39 L0
